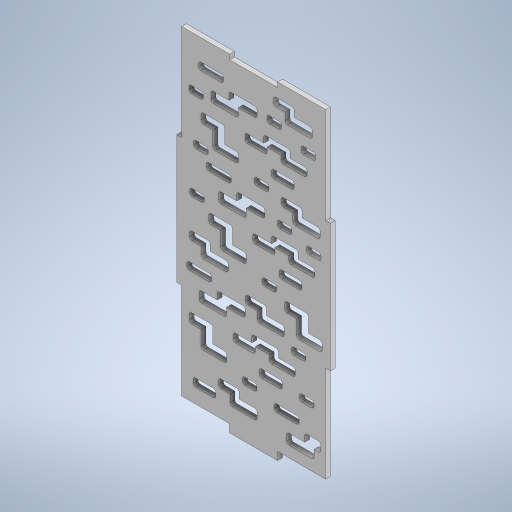
# Autodesk Inventor part: Pièce Ve3
Saved by Autodesk Inventor 2023 (Build 270158000, 158)
## iProperties
Created: 2025-01-14
Part Number: Pièce Ve3
Material: Générique
Document SubType Name: Modeling
Designer: kfadieieva
Density: 1 g/cm^3
Appearance: Par défaut
Author: kfadieieva
Autodesk Inventor part; units mm, degrees
ref_plane "YZ Plane" through (0, 0, 0) normal (1, 0, 0) x (0, 1, 0)
ref_plane "XZ Plane" through (0, 0, 0) normal (0, 1, 0) x (-1, 0, 0)
ref_plane "XY Plane" through (0, 0, 0) normal (0, 0, 1) x (1, 0, 0)
sketch "Esquisse1" plane through (0, 0, 0) normal (0, 0, 1) x (1, 0, 0)
  line L0 (96, 60) -> (96, 139.9775)
  line L1 (0, 140) -> (0, 60)
  line L2 (33, 199.9775) -> (33, 196.9775)
  line L3 (33, 196.9775) -> (63, 196.9775)
  line L4 (63, 196.9775) -> (63, 199.9775)
  line L5 (96, 139.9775) -> (93, 139.9775)
  line L6 (93, 139.9775) -> (93, 199.9775)
  line L7 (96, 60) -> (93, 60)
  line L8 (0, 60) -> (3, 60)
  line L9 (3, 60) -> (3, 0)
  line L10 (0, 140) -> (3, 140)
  line L11 (3, 140) -> (3, 199.9775)
  line L12 (93, 199.9775) -> (63, 199.9775)
  line L13 (33, 199.9775) -> (3, 199.9775)
  line L14 (63, -5) -> (33, -5)
  line L15 (33, -5) -> (33, 0)
  line L16 (3, 0) -> (33, 0)
  line L17 (63, -5) -> (63, 0)
  line L18 (63, 0) -> (93, 0)
  line L19 (93, 0) -> (93, 60)
  point P0 (0, 0)
  point P1 (18, 199.9775)
  dimension "d2" = 33
  dimension "d3" = 33
  dimension "d6" = 3
  dimension "d7" = 3
  dimension "d8" = 3
  dimension "d9" = 3
  dimension "d25" = 33
  dimension "d27" = 60
  dimension "d28" = 90
  dimension "d29" = 90
  dimension "d30" = 90
  dimension "d31" = 90
  dimension "d34" = 90
  dimension "d35" = 90
  dimension "d36" = 90
  dimension "d37" = 90
  dimension "d38" = 90
  dimension "d39" = 5
  dimension "d41" = 90
  dimension "d42" = 90
  dimension "d43" = 90
  dimension "d44" = 96
  dimension "d45" = 199.9775
  constraints: 40 end point, 11 perpendicular, 3 horizontal, 3 parallel, 2 point on line, 2 vertical, 1 midpoint
  measures "d2" distance from line of L0 L4.end
  measures "d3" distance from line of L1 L2.start
  measures "d6" distance of L0.end L5.end
  measures "d7" distance of L1.start L10.end
  measures "d8" distance of L1.end L8.end
  measures "d9" distance of L3.end L4.end
  measures "d25" distance between parallel lines of L15 L1
  measures "d27" distance of L8.end L9.end
  measures "d28" angle of L13 L11
  measures "d29" angle of L2 L13
  measures "d30" angle of L12 L4
  measures "d31" angle of L6 L12
  measures "d34" angle of L16 L9
  measures "d35" angle of L1 L8
  measures "d36" angle of L9 L8
  measures "d37" angle of L10 L1
  measures "d38" angle of L6 L5
  measures "d39" distance of L14.end L15.end
  measures "d41" angle of L14 L15
  measures "d42" angle of L15 L16
  measures "d43" angle of L0 L7
  measures "d44" distance between parallel lines of L0 L1
  measures "d45" distance between parallel lines of L18 L12
extrude "Extrusion1" add sketch "Esquisse1" along normal blind 3
sketch "Esquisse3" plane through (0, 0, 3) normal (0, 0, 1) x (1, 0, 0)
  line L0 (15.2322, 186.7722) -> (27.611, 186.7722)
  line L1 (29.111, 185.2722) -> (29.111, 183.7396)
  line L2 (27.611, 182.2396) -> (15.2322, 182.2396)
  line L3 (13.7322, 183.7396) -> (13.7322, 185.2722)
  line L4 (22.9216, 174.793) -> (32.6723, 174.793)
  line L5 (38.5001, 173.8217) -> (38.5001, 169.8178)
  line L6 (37.0001, 168.3178) -> (22.9216, 168.3178)
  line L7 (21.4216, 169.8178) -> (21.4216, 173.293)
  line L8 (34.1723, 179.8113) -> (48.6555, 179.8113)
  line L9 (50.1555, 178.3113) -> (50.1555, 175.3217)
  line L10 (48.6555, 173.8217) -> (38.5001, 173.8217)
  line L11 (32.6723, 174.793) -> (32.6723, 178.3113)
  line L12 (62.016, 191.143) -> (71.9234, 191.143)
  line L13 (73.4234, 189.643) -> (73.4234, 185.9628)
  line L14 (67.7197, 185.9628) -> (62.016, 185.9628)
  line L15 (60.516, 187.4628) -> (60.516, 189.643)
  line L16 (73.4234, 185.9628) -> (83.1363, 185.9628)
  line L17 (84.6363, 184.4628) -> (84.6363, 181.3113)
  line L18 (83.1363, 179.8113) -> (69.2197, 179.8113)
  line L19 (67.7197, 181.3113) -> (67.7197, 185.9628)
  line L20 (55.8645, 167.1846) -> (69.3764, 167.1846)
  line L21 (70.8764, 165.6846) -> (70.8764, 162.49)
  line L22 (65.2105, 161.5187) -> (56.4689, 161.5187)
  line L23 (54.3645, 162.49) -> (54.3645, 165.6846)
  line L24 (70.8764, 162.49) -> (79.8987, 162.49)
  line L25 (81.3987, 160.99) -> (81.3987, 158.8098)
  line L26 (79.8987, 157.3098) -> (66.7105, 157.3098)
  line L27 (65.2105, 158.8098) -> (65.2105, 161.5187)
  line L28 (44.209, 162.49) -> (54.3645, 162.49)
  line L29 (56.4689, 161.5187) -> (56.4689, 158.8098)
  line L30 (54.9689, 157.3098) -> (44.209, 157.3098)
  line L31 (42.709, 158.8098) -> (42.709, 160.99)
  line L32 (16.6892, 159.8999) -> (28.4608, 159.8999)
  line L33 (29.9608, 158.3999) -> (29.9608, 153.9103)
  line L34 (22.575, 153.9103) -> (16.6892, 153.9103)
  line L35 (15.1892, 155.4103) -> (15.1892, 158.3999)
  line L36 (29.9608, 155.5291) -> (29.9608, 149.5395)
  line L37 (22.575, 147.2732) -> (22.575, 153.9103)
  line L38 (29.9608, 149.5395) -> (37.0001, 149.5395)
  line L39 (38.5001, 148.0395) -> (38.5001, 144.888)
  line L40 (37.0001, 143.388) -> (24.075, 143.388)
  line L41 (22.575, 144.888) -> (22.575, 149.5395)
  line L42 (60.7209, 151.4012) -> (71.8046, 151.4012)
  line L43 (73.3046, 149.9012) -> (73.3046, 147.9638)
  line L44 (71.8046, 146.4638) -> (60.7209, 146.4638)
  line L45 (59.2209, 147.9638) -> (59.2209, 149.9012)
  line L46 (50.0075, 141.672) -> (55.9505, 141.672)
  line L47 (57.4505, 140.172) -> (57.4505, 138.8448)
  line L48 (55.9505, 137.3448) -> (50.0075, 137.3448)
  line L49 (48.5075, 138.8448) -> (48.5075, 140.172)
  arc A0 (15.2322, 186.7722) -> (13.7322, 185.2722) centre (15.2322, 185.2722) ccw
  arc A1 (13.7322, 183.7396) -> (15.2322, 182.2396) centre (15.2322, 183.7396) ccw
  arc A2 (29.111, 185.2722) -> (27.611, 186.7722) centre (27.611, 185.2722) ccw
  arc A3 (27.611, 182.2396) -> (29.111, 183.7396) centre (27.611, 183.7396) ccw
  arc A4 (34.1723, 179.8113) -> (32.6723, 178.3113) centre (34.1723, 178.3113) ccw
  arc A5 (22.9216, 174.793) -> (21.4216, 173.293) centre (22.9216, 173.293) ccw
  arc A6 (21.4216, 169.8178) -> (22.9216, 168.3178) centre (22.9216, 169.8178) ccw
  arc A7 (37.0001, 168.3178) -> (38.5001, 169.8178) centre (37.0001, 169.8178) ccw
  arc A8 (50.1555, 178.3113) -> (48.6555, 179.8113) centre (48.6555, 178.3113) ccw
  arc A9 (48.6555, 173.8217) -> (50.1555, 175.3217) centre (48.6555, 175.3217) ccw
  arc A10 (60.516, 187.4628) -> (62.016, 185.9628) centre (62.016, 187.4628) ccw
  arc A11 (62.016, 191.143) -> (60.516, 189.643) centre (62.016, 189.643) ccw
  arc A12 (73.4234, 189.643) -> (71.9234, 191.143) centre (71.9234, 189.643) ccw
  arc A13 (83.1363, 179.8113) -> (84.6363, 181.3113) centre (83.1363, 181.3113) ccw
  arc A14 (84.6363, 184.4628) -> (83.1363, 185.9628) centre (83.1363, 184.4628) ccw
  arc A15 (67.7197, 181.3113) -> (69.2197, 179.8113) centre (69.2197, 181.3113) ccw
  arc A16 (70.8764, 165.6846) -> (69.3764, 167.1846) centre (69.3764, 165.6846) ccw
  arc A17 (65.2105, 158.8098) -> (66.7105, 157.3098) centre (66.7105, 158.8098) ccw
  arc A18 (81.3987, 160.99) -> (79.8987, 162.49) centre (79.8987, 160.99) ccw
  arc A19 (79.8987, 157.3098) -> (81.3987, 158.8098) centre (79.8987, 158.8098) ccw
  arc A20 (55.8645, 167.1846) -> (54.3645, 165.6846) centre (55.8645, 165.6846) ccw
  arc A21 (44.209, 162.49) -> (42.709, 160.99) centre (44.209, 160.99) ccw
  arc A22 (42.709, 158.8098) -> (44.209, 157.3098) centre (44.209, 158.8098) ccw
  arc A23 (54.9689, 157.3098) -> (56.4689, 158.8098) centre (54.9689, 158.8098) ccw
  arc A24 (60.7209, 151.4012) -> (59.2209, 149.9012) centre (60.7209, 149.9012) ccw
  arc A25 (59.2209, 147.9638) -> (60.7209, 146.4638) centre (60.7209, 147.9638) ccw
  arc A26 (71.8046, 146.4638) -> (73.3046, 147.9638) centre (71.8046, 147.9638) ccw
  arc A27 (73.3046, 149.9012) -> (71.8046, 151.4012) centre (71.8046, 149.9012) ccw
  arc A28 (57.4505, 140.172) -> (55.9505, 141.672) centre (55.9505, 140.172) ccw
  arc A29 (55.9505, 137.3448) -> (57.4505, 138.8448) centre (55.9505, 138.8448) ccw
  arc A30 (48.5075, 138.8448) -> (50.0075, 137.3448) centre (50.0075, 138.8448) ccw
  arc A31 (50.0075, 141.672) -> (48.5075, 140.172) centre (50.0075, 140.172) ccw
  arc A32 (37.0001, 143.388) -> (38.5001, 144.888) centre (37.0001, 144.888) ccw
  arc A33 (38.5001, 148.0395) -> (37.0001, 149.5395) centre (37.0001, 148.0395) ccw
  arc A34 (22.575, 144.888) -> (24.075, 143.388) centre (24.075, 144.888) ccw
  arc A35 (15.1892, 155.4103) -> (16.6892, 153.9103) centre (16.6892, 155.4103) ccw
  arc A36 (16.6892, 159.8999) -> (15.1892, 158.3999) centre (16.6892, 158.3999) ccw
  arc A37 (29.9608, 158.3999) -> (28.4608, 159.8999) centre (28.4608, 158.3999) ccw
  line L50 (20.1228, 134.7776) -> (32.5015, 134.7776)
  line L51 (34.0015, 133.2776) -> (34.0015, 131.7449)
  line L52 (32.5015, 130.2449) -> (20.1228, 130.2449)
  line L53 (18.6228, 131.7449) -> (18.6228, 133.2776)
  line L54 (27.8122, 122.7984) -> (37.5629, 122.7984)
  line L55 (43.3907, 121.8271) -> (43.3907, 117.8231)
  line L56 (41.8907, 116.3231) -> (27.8122, 116.3231)
  line L57 (26.3122, 117.8231) -> (26.3122, 121.2984)
  line L58 (39.0629, 127.8167) -> (53.5461, 127.8167)
  line L59 (55.0461, 126.3167) -> (55.0461, 123.3271)
  line L60 (53.5461, 121.8271) -> (43.3907, 121.8271)
  line L61 (37.5629, 122.7984) -> (37.5629, 126.3167)
  line L62 (66.9065, 139.1484) -> (76.814, 139.1484)
  line L63 (78.314, 137.6484) -> (78.314, 133.9682)
  line L64 (72.6103, 133.9682) -> (66.9065, 133.9682)
  line L65 (65.4065, 135.4682) -> (65.4065, 137.6484)
  line L66 (78.314, 133.9682) -> (88.0269, 133.9682)
  line L67 (89.5269, 132.4682) -> (89.5269, 129.3167)
  line L68 (88.0269, 127.8167) -> (74.1103, 127.8167)
  line L69 (72.6103, 129.3167) -> (72.6103, 133.9682)
  line L70 (60.7551, 115.1899) -> (74.267, 115.1899)
  line L71 (75.767, 113.6899) -> (75.767, 110.4954)
  line L72 (70.1011, 109.5241) -> (61.3595, 109.5241)
  line L73 (59.2551, 110.4954) -> (59.2551, 113.6899)
  line L74 (75.767, 110.4954) -> (84.7893, 110.4954)
  line L75 (86.2893, 108.9954) -> (86.2893, 106.8152)
  line L76 (84.7893, 105.3152) -> (71.6011, 105.3152)
  line L77 (70.1011, 106.8152) -> (70.1011, 109.5241)
  line L78 (49.0996, 110.4954) -> (59.2551, 110.4954)
  line L79 (61.3595, 109.5241) -> (61.3595, 106.8152)
  line L80 (59.8595, 105.3152) -> (49.0996, 105.3152)
  line L81 (47.5996, 106.8152) -> (47.5996, 108.9954)
  line L82 (21.5797, 107.9053) -> (33.3514, 107.9053)
  line L83 (34.8514, 106.4053) -> (34.8514, 101.9156)
  line L84 (27.4656, 101.9156) -> (21.5797, 101.9156)
  line L85 (20.0797, 103.4156) -> (20.0797, 106.4053)
  line L86 (34.8514, 103.5345) -> (34.8514, 97.5448)
  line L87 (27.4656, 95.2785) -> (27.4656, 101.9156)
  line L88 (34.8514, 97.5448) -> (41.8907, 97.5448)
  line L89 (43.3907, 96.0448) -> (43.3907, 92.8933)
  line L90 (41.8907, 91.3933) -> (28.9656, 91.3933)
  line L91 (27.4656, 92.8933) -> (27.4656, 97.5448)
  line L92 (65.6115, 99.4065) -> (76.6952, 99.4065)
  line L93 (78.1952, 97.9065) -> (78.1952, 95.9691)
  line L94 (76.6952, 94.4691) -> (65.6115, 94.4691)
  line L95 (64.1115, 95.9691) -> (64.1115, 97.9065)
  line L96 (54.8981, 89.6774) -> (60.8411, 89.6774)
  line L97 (62.3411, 88.1774) -> (62.3411, 86.8501)
  line L98 (60.8411, 85.3501) -> (54.8981, 85.3501)
  line L99 (53.3981, 86.8501) -> (53.3981, 88.1774)
  arc A38 (20.1228, 134.7776) -> (18.6228, 133.2776) centre (20.1228, 133.2776) ccw
  arc A39 (18.6228, 131.7449) -> (20.1228, 130.2449) centre (20.1228, 131.7449) ccw
  arc A40 (34.0015, 133.2776) -> (32.5015, 134.7776) centre (32.5015, 133.2776) ccw
  arc A41 (32.5015, 130.2449) -> (34.0015, 131.7449) centre (32.5015, 131.7449) ccw
  arc A42 (39.0629, 127.8167) -> (37.5629, 126.3167) centre (39.0629, 126.3167) ccw
  arc A43 (27.8122, 122.7984) -> (26.3122, 121.2984) centre (27.8122, 121.2984) ccw
  arc A44 (26.3122, 117.8231) -> (27.8122, 116.3231) centre (27.8122, 117.8231) ccw
  arc A45 (41.8907, 116.3231) -> (43.3907, 117.8231) centre (41.8907, 117.8231) ccw
  arc A46 (55.0461, 126.3167) -> (53.5461, 127.8167) centre (53.5461, 126.3167) ccw
  arc A47 (53.5461, 121.8271) -> (55.0461, 123.3271) centre (53.5461, 123.3271) ccw
  arc A48 (65.4065, 135.4682) -> (66.9065, 133.9682) centre (66.9065, 135.4682) ccw
  arc A49 (66.9065, 139.1484) -> (65.4065, 137.6484) centre (66.9065, 137.6484) ccw
  arc A50 (78.314, 137.6484) -> (76.814, 139.1484) centre (76.814, 137.6484) ccw
  arc A51 (88.0269, 127.8167) -> (89.5269, 129.3167) centre (88.0269, 129.3167) ccw
  arc A52 (89.5269, 132.4682) -> (88.0269, 133.9682) centre (88.0269, 132.4682) ccw
  arc A53 (72.6103, 129.3167) -> (74.1103, 127.8167) centre (74.1103, 129.3167) ccw
  arc A54 (75.767, 113.6899) -> (74.267, 115.1899) centre (74.267, 113.6899) ccw
  arc A55 (70.1011, 106.8152) -> (71.6011, 105.3152) centre (71.6011, 106.8152) ccw
  arc A56 (86.2893, 108.9954) -> (84.7893, 110.4954) centre (84.7893, 108.9954) ccw
  arc A57 (84.7893, 105.3152) -> (86.2893, 106.8152) centre (84.7893, 106.8152) ccw
  arc A58 (60.7551, 115.1899) -> (59.2551, 113.6899) centre (60.7551, 113.6899) ccw
  arc A59 (49.0996, 110.4954) -> (47.5996, 108.9954) centre (49.0996, 108.9954) ccw
  arc A60 (47.5996, 106.8152) -> (49.0996, 105.3152) centre (49.0996, 106.8152) ccw
  arc A61 (59.8595, 105.3152) -> (61.3595, 106.8152) centre (59.8595, 106.8152) ccw
  arc A62 (65.6115, 99.4065) -> (64.1115, 97.9065) centre (65.6115, 97.9065) ccw
  arc A63 (64.1115, 95.9691) -> (65.6115, 94.4691) centre (65.6115, 95.9691) ccw
  arc A64 (76.6952, 94.4691) -> (78.1952, 95.9691) centre (76.6952, 95.9691) ccw
  arc A65 (78.1952, 97.9065) -> (76.6952, 99.4065) centre (76.6952, 97.9065) ccw
  arc A66 (62.3411, 88.1774) -> (60.8411, 89.6774) centre (60.8411, 88.1774) ccw
  arc A67 (60.8411, 85.3501) -> (62.3411, 86.8501) centre (60.8411, 86.8501) ccw
  arc A68 (53.3981, 86.8501) -> (54.8981, 85.3501) centre (54.8981, 86.8501) ccw
  arc A69 (54.8981, 89.6774) -> (53.3981, 88.1774) centre (54.8981, 88.1774) ccw
  arc A70 (41.8907, 91.3933) -> (43.3907, 92.8933) centre (41.8907, 92.8933) ccw
  arc A71 (43.3907, 96.0448) -> (41.8907, 97.5448) centre (41.8907, 96.0448) ccw
  arc A72 (27.4656, 92.8933) -> (28.9656, 91.3933) centre (28.9656, 92.8933) ccw
  arc A73 (20.0797, 103.4156) -> (21.5797, 101.9156) centre (21.5797, 103.4156) ccw
  arc A74 (21.5797, 107.9053) -> (20.0797, 106.4053) centre (21.5797, 106.4053) ccw
  arc A75 (34.8514, 106.4053) -> (33.3514, 107.9053) centre (33.3514, 106.4053) ccw
  line L100 (7.859, 75.0609) -> (20.2378, 75.0609)
  line L101 (21.7378, 73.5609) -> (21.7378, 72.0282)
  line L102 (20.2378, 70.5282) -> (7.859, 70.5282)
  line L103 (6.359, 72.0282) -> (6.359, 73.5609)
  line L104 (15.5484, 63.0817) -> (25.2992, 63.0817)
  line L105 (31.1269, 62.1104) -> (31.1269, 58.1064)
  line L106 (29.6269, 56.6064) -> (15.5484, 56.6064)
  line L107 (14.0484, 58.1064) -> (14.0484, 61.5817)
  line L108 (26.7992, 68.1) -> (41.2824, 68.1)
  line L109 (42.7824, 66.6) -> (42.7824, 63.6104)
  line L110 (41.2824, 62.1104) -> (31.1269, 62.1104)
  line L111 (25.2992, 63.0817) -> (25.2992, 66.6)
  line L112 (44.5787, 75.1578) -> (54.4861, 75.1578)
  line L113 (55.9861, 73.6578) -> (55.9861, 69.9776)
  line L114 (50.2824, 69.9776) -> (44.5787, 69.9776)
  line L115 (43.0787, 71.4776) -> (43.0787, 73.6578)
  line L116 (55.9861, 69.9776) -> (65.699, 69.9776)
  line L117 (67.199, 68.4776) -> (67.199, 65.3261)
  line L118 (65.699, 63.8261) -> (51.7824, 63.8261)
  line L119 (50.2824, 65.3261) -> (50.2824, 69.9776)
  line L120 (48.4913, 55.4733) -> (62.0032, 55.4733)
  line L121 (63.5032, 53.9733) -> (63.5032, 50.7787)
  line L122 (57.8373, 49.8074) -> (49.0957, 49.8074)
  line L123 (46.9913, 50.7787) -> (46.9913, 53.9733)
  line L124 (63.5032, 50.7787) -> (72.5255, 50.7787)
  line L125 (74.0255, 49.2787) -> (74.0255, 47.0985)
  line L126 (72.5255, 45.5985) -> (59.3373, 45.5985)
  line L127 (57.8373, 47.0985) -> (57.8373, 49.8074)
  line L128 (36.8358, 50.7787) -> (46.9913, 50.7787)
  line L129 (49.0957, 49.8074) -> (49.0957, 47.0985)
  line L130 (47.5957, 45.5985) -> (36.8358, 45.5985)
  line L131 (35.3358, 47.0985) -> (35.3358, 49.2787)
  line L132 (9.316, 48.1886) -> (21.0877, 48.1886)
  line L133 (22.5877, 46.6886) -> (22.5877, 42.199)
  line L134 (15.2018, 42.199) -> (9.316, 42.199)
  line L135 (7.816, 43.699) -> (7.816, 46.6886)
  line L136 (22.5877, 43.8178) -> (22.5877, 37.8282)
  line L137 (15.2018, 35.5619) -> (15.2018, 42.199)
  line L138 (22.5877, 37.8282) -> (29.6269, 37.8282)
  line L139 (31.1269, 36.3282) -> (31.1269, 33.1767)
  line L140 (29.6269, 31.6767) -> (16.7018, 31.6767)
  line L141 (15.2018, 33.1767) -> (15.2018, 37.8282)
  line L142 (53.3477, 39.6898) -> (64.4314, 39.6898)
  line L143 (65.9314, 38.1898) -> (65.9314, 36.2524)
  line L144 (64.4314, 34.7524) -> (53.3477, 34.7524)
  line L145 (51.8477, 36.2524) -> (51.8477, 38.1898)
  line L146 (42.6343, 29.9607) -> (48.5773, 29.9607)
  line L147 (50.0773, 28.4607) -> (50.0773, 27.1335)
  line L148 (48.5773, 25.6335) -> (42.6343, 25.6335)
  line L149 (41.1343, 27.1335) -> (41.1343, 28.4607)
  arc A76 (7.859, 75.0609) -> (6.359, 73.5609) centre (7.859, 73.5609) ccw
  arc A77 (6.359, 72.0282) -> (7.859, 70.5282) centre (7.859, 72.0282) ccw
  arc A78 (21.7378, 73.5609) -> (20.2378, 75.0609) centre (20.2378, 73.5609) ccw
  arc A79 (20.2378, 70.5282) -> (21.7378, 72.0282) centre (20.2378, 72.0282) ccw
  arc A80 (26.7992, 68.1) -> (25.2992, 66.6) centre (26.7992, 66.6) ccw
  arc A81 (15.5484, 63.0817) -> (14.0484, 61.5817) centre (15.5484, 61.5817) ccw
  arc A82 (14.0484, 58.1064) -> (15.5484, 56.6064) centre (15.5484, 58.1064) ccw
  arc A83 (29.6269, 56.6064) -> (31.1269, 58.1064) centre (29.6269, 58.1064) ccw
  arc A84 (42.7824, 66.6) -> (41.2824, 68.1) centre (41.2824, 66.6) ccw
  arc A85 (41.2824, 62.1104) -> (42.7824, 63.6104) centre (41.2824, 63.6104) ccw
  arc A86 (43.0787, 71.4776) -> (44.5787, 69.9776) centre (44.5787, 71.4776) ccw
  arc A87 (44.5787, 75.1578) -> (43.0787, 73.6578) centre (44.5787, 73.6578) ccw
  arc A88 (55.9861, 73.6578) -> (54.4861, 75.1578) centre (54.4861, 73.6578) ccw
  arc A89 (65.699, 63.8261) -> (67.199, 65.3261) centre (65.699, 65.3261) ccw
  arc A90 (67.199, 68.4776) -> (65.699, 69.9776) centre (65.699, 68.4776) ccw
  arc A91 (50.2824, 65.3261) -> (51.7824, 63.8261) centre (51.7824, 65.3261) ccw
  arc A92 (63.5032, 53.9733) -> (62.0032, 55.4733) centre (62.0032, 53.9733) ccw
  arc A93 (57.8373, 47.0985) -> (59.3373, 45.5985) centre (59.3373, 47.0985) ccw
  arc A94 (74.0255, 49.2787) -> (72.5255, 50.7787) centre (72.5255, 49.2787) ccw
  arc A95 (72.5255, 45.5985) -> (74.0255, 47.0985) centre (72.5255, 47.0985) ccw
  arc A96 (48.4913, 55.4733) -> (46.9913, 53.9733) centre (48.4913, 53.9733) ccw
  arc A97 (36.8358, 50.7787) -> (35.3358, 49.2787) centre (36.8358, 49.2787) ccw
  arc A98 (35.3358, 47.0985) -> (36.8358, 45.5985) centre (36.8358, 47.0985) ccw
  arc A99 (47.5957, 45.5985) -> (49.0957, 47.0985) centre (47.5957, 47.0985) ccw
  arc A100 (53.3477, 39.6898) -> (51.8477, 38.1898) centre (53.3477, 38.1898) ccw
  arc A101 (51.8477, 36.2524) -> (53.3477, 34.7524) centre (53.3477, 36.2524) ccw
  arc A102 (64.4314, 34.7524) -> (65.9314, 36.2524) centre (64.4314, 36.2524) ccw
  arc A103 (65.9314, 38.1898) -> (64.4314, 39.6898) centre (64.4314, 38.1898) ccw
  arc A104 (50.0773, 28.4607) -> (48.5773, 29.9607) centre (48.5773, 28.4607) ccw
  arc A105 (48.5773, 25.6335) -> (50.0773, 27.1335) centre (48.5773, 27.1335) ccw
  arc A106 (41.1343, 27.1335) -> (42.6343, 25.6335) centre (42.6343, 27.1335) ccw
  arc A107 (42.6343, 29.9607) -> (41.1343, 28.4607) centre (42.6343, 28.4607) ccw
  arc A108 (29.6269, 31.6767) -> (31.1269, 33.1767) centre (29.6269, 33.1767) ccw
  arc A109 (31.1269, 36.3282) -> (29.6269, 37.8282) centre (29.6269, 36.3282) ccw
  arc A110 (15.2018, 33.1767) -> (16.7018, 31.6767) centre (16.7018, 33.1767) ccw
  arc A111 (7.816, 43.699) -> (9.316, 42.199) centre (9.316, 43.699) ccw
  arc A112 (9.316, 48.1886) -> (7.816, 46.6886) centre (9.316, 46.6886) ccw
  arc A113 (22.5877, 46.6886) -> (21.0877, 48.1886) centre (21.0877, 46.6886) ccw
  line L150 (62.5345, 25.4266) -> (74.9132, 25.4266)
  line L151 (76.4132, 23.9266) -> (76.4132, 22.3939)
  line L152 (74.9132, 20.8939) -> (62.5345, 20.8939)
  line L153 (61.0345, 22.3939) -> (61.0345, 23.9266)
  line L154 (70.2239, 13.4474) -> (79.9746, 13.4474)
  line L155 (85.8024, 12.4761) -> (85.8024, 8.4721)
  line L156 (84.3024, 6.9721) -> (70.2239, 6.9721)
  line L157 (68.7239, 8.4721) -> (68.7239, 11.9474)
  line L158 (79.9746, 13.4474) -> (79.9746, 16.9657)
  line L159 (9.5387, 92.4703) -> (19.4461, 92.4703)
  line L160 (20.9461, 90.9703) -> (20.9461, 87.2901)
  line L161 (15.2424, 87.2901) -> (9.5387, 87.2901)
  line L162 (8.0387, 88.7901) -> (8.0387, 90.9703)
  line L163 (20.9461, 87.2901) -> (30.659, 87.2901)
  line L164 (32.159, 85.7901) -> (32.159, 82.6386)
  line L165 (30.659, 81.1386) -> (16.7424, 81.1386)
  line L166 (15.2424, 82.6386) -> (15.2424, 87.2901)
  line L167 (69.0763, 83.9073) -> (80.848, 83.9073)
  line L168 (82.348, 82.4073) -> (82.348, 77.9177)
  line L169 (74.9621, 77.9177) -> (69.0763, 77.9177)
  line L170 (67.5763, 79.4177) -> (67.5763, 82.4073)
  line L171 (82.348, 79.5365) -> (82.348, 73.5469)
  line L172 (74.9621, 71.2806) -> (74.9621, 77.9177)
  line L173 (82.348, 73.5469) -> (89.3872, 73.5469)
  line L174 (90.8872, 72.0469) -> (90.8872, 68.8954)
  line L175 (89.3872, 67.3954) -> (76.4621, 67.3954)
  line L176 (74.9621, 68.8954) -> (74.9621, 73.5469)
  line L177 (11.7943, 14.1137) -> (22.878, 14.1137)
  line L178 (24.378, 12.6137) -> (24.378, 10.6763)
  line L179 (22.878, 9.1763) -> (11.7943, 9.1763)
  line L180 (10.2943, 10.6763) -> (10.2943, 12.6137)
  line L181 (78.3166, 38.6119) -> (84.2595, 38.6119)
  line L182 (85.7595, 37.1119) -> (85.7595, 35.7846)
  line L183 (84.2595, 34.2846) -> (78.3166, 34.2846)
  line L184 (76.8166, 35.7846) -> (76.8166, 37.1119)
  arc A114 (62.5345, 25.4266) -> (61.0345, 23.9266) centre (62.5345, 23.9266) ccw
  arc A115 (61.0345, 22.3939) -> (62.5345, 20.8939) centre (62.5345, 22.3939) ccw
  arc A116 (76.4132, 23.9266) -> (74.9132, 25.4266) centre (74.9132, 23.9266) ccw
  arc A117 (74.9132, 20.8939) -> (76.4132, 22.3939) centre (74.9132, 22.3939) ccw
  arc A118 (81.4746, 18.4657) -> (79.9746, 16.9657) centre (81.4746, 16.9657) ccw
  arc A119 (70.2239, 13.4474) -> (68.7239, 11.9474) centre (70.2239, 11.9474) ccw
  arc A120 (68.7239, 8.4721) -> (70.2239, 6.9721) centre (70.2239, 8.4721) ccw
  arc A121 (84.3024, 6.9721) -> (85.8024, 8.4721) centre (84.3024, 8.4721) ccw
  arc A122 (8.0387, 88.7901) -> (9.5387, 87.2901) centre (9.5387, 88.7901) ccw
  arc A123 (9.5387, 92.4703) -> (8.0387, 90.9703) centre (9.5387, 90.9703) ccw
  arc A124 (20.9461, 90.9703) -> (19.4461, 92.4703) centre (19.4461, 90.9703) ccw
  arc A125 (30.659, 81.1386) -> (32.159, 82.6386) centre (30.659, 82.6386) ccw
  arc A126 (32.159, 85.7901) -> (30.659, 87.2901) centre (30.659, 85.7901) ccw
  arc A127 (15.2424, 82.6386) -> (16.7424, 81.1386) centre (16.7424, 82.6386) ccw
  arc A128 (11.7943, 14.1137) -> (10.2943, 12.6137) centre (11.7943, 12.6137) ccw
  arc A129 (10.2943, 10.6763) -> (11.7943, 9.1763) centre (11.7943, 10.6763) ccw
  arc A130 (22.878, 9.1763) -> (24.378, 10.6763) centre (22.878, 10.6763) ccw
  arc A131 (24.378, 12.6137) -> (22.878, 14.1137) centre (22.878, 12.6137) ccw
  arc A132 (85.7595, 37.1119) -> (84.2595, 38.6119) centre (84.2595, 37.1119) ccw
  arc A133 (84.2595, 34.2846) -> (85.7595, 35.7846) centre (84.2595, 35.7846) ccw
  arc A134 (76.8166, 35.7846) -> (78.3166, 34.2846) centre (78.3166, 35.7846) ccw
  arc A135 (78.3166, 38.6119) -> (76.8166, 37.1119) centre (78.3166, 37.1119) ccw
  arc A136 (89.3872, 67.3954) -> (90.8872, 68.8954) centre (89.3872, 68.8954) ccw
  arc A137 (90.8872, 72.0469) -> (89.3872, 73.5469) centre (89.3872, 72.0469) ccw
  arc A138 (74.9621, 68.8954) -> (76.4621, 67.3954) centre (76.4621, 68.8954) ccw
  arc A139 (67.5763, 79.4177) -> (69.0763, 77.9177) centre (69.0763, 79.4177) ccw
  arc A140 (69.0763, 83.9073) -> (67.5763, 82.4073) centre (69.0763, 82.4073) ccw
  arc A141 (82.348, 82.4073) -> (80.848, 83.9073) centre (80.848, 82.4073) ccw
  line L185 (27.6073, 21.4563) -> (37.5148, 21.4563)
  line L186 (39.0148, 19.9563) -> (39.0148, 16.2761)
  line L187 (33.3111, 16.2761) -> (27.6073, 16.2761)
  line L188 (26.1073, 17.7761) -> (26.1073, 19.9563)
  line L189 (39.0148, 16.2761) -> (48.7277, 16.2761)
  line L190 (50.2277, 14.7761) -> (50.2277, 11.6246)
  line L191 (48.7277, 10.1246) -> (34.8111, 10.1246)
  line L192 (33.3111, 11.6246) -> (33.3111, 16.2761)
  line L193 (9.6709, 115.6112) -> (15.6139, 115.6112)
  line L194 (17.1139, 114.1112) -> (17.1139, 112.784)
  line L195 (15.6139, 111.284) -> (9.6709, 111.284)
  line L196 (8.1709, 112.784) -> (8.1709, 114.1112)
  arc A142 (-19.1764, 17.0855) -> (-19.2195, 17.0849) centre (-19.1764, 15.5855) ccw
  arc A143 (26.1073, 17.7761) -> (27.6073, 16.2761) centre (27.6073, 17.7761) ccw
  arc A144 (27.6073, 21.4563) -> (26.1073, 19.9563) centre (27.6073, 19.9563) ccw
  arc A145 (39.0148, 19.9563) -> (37.5148, 21.4563) centre (37.5148, 19.9563) ccw
  arc A146 (48.7277, 10.1246) -> (50.2277, 11.6246) centre (48.7277, 11.6246) ccw
  arc A147 (50.2277, 14.7761) -> (48.7277, 16.2761) centre (48.7277, 14.7761) ccw
  arc A148 (33.3111, 11.6246) -> (34.8111, 10.1246) centre (34.8111, 11.6246) ccw
  arc A149 (17.1139, 114.1112) -> (15.6139, 115.6112) centre (15.6139, 114.1112) ccw
  arc A150 (15.6139, 111.284) -> (17.1139, 112.784) centre (15.6139, 112.784) ccw
  arc A151 (8.1709, 112.784) -> (9.6709, 111.284) centre (9.6709, 112.784) ccw
  arc A152 (9.6709, 115.6112) -> (8.1709, 114.1112) centre (9.6709, 114.1112) ccw
  line L197 (88.5113, 12.4761) -> (85.8024, 12.4761)
  line L198 (81.4746, 18.4657) -> (88.5113, 18.4657)
  line L199 (90.0113, 16.9657) -> (90.0113, 13.9761)
  arc A153 (88.5113, 12.4761) -> (90.0113, 13.9761) centre (88.5113, 13.9761) ccw
  arc A154 (90.0113, 16.9657) -> (88.5113, 18.4657) centre (88.5113, 16.9657) ccw
  line L200 (64.4612, 125.6561) -> (70.4042, 125.6561)
  arc A155 (71.9042, 124.1561) -> (70.4042, 125.6561) centre (70.4042, 124.1561) ccw
  arc A156 (64.4612, 125.6561) -> (62.9612, 124.1561) centre (64.4612, 124.1561) ccw
  line L201 (71.9042, 124.1561) -> (71.9042, 122.8289)
  arc A157 (62.9612, 122.8289) -> (64.4612, 121.3289) centre (64.4612, 122.8289) ccw
  line L202 (70.4042, 121.3289) -> (64.4612, 121.3289)
  arc A158 (70.4042, 121.3289) -> (71.9042, 122.8289) centre (70.4042, 122.8289) ccw
  line L203 (62.9612, 122.8289) -> (62.9612, 124.1561)
  line L204 (82.6873, 120.6683) -> (88.6303, 120.6683)
  arc A159 (90.1303, 119.1683) -> (88.6303, 120.6683) centre (88.6303, 119.1683) ccw
  arc A160 (82.6873, 120.6683) -> (81.1873, 119.1683) centre (82.6873, 119.1683) ccw
  line L205 (90.1303, 119.1683) -> (90.1303, 117.8411)
  arc A161 (81.1873, 117.8411) -> (82.6873, 116.3411) centre (82.6873, 117.8411) ccw
  line L206 (88.6303, 116.3411) -> (82.6873, 116.3411)
  arc A162 (88.6303, 116.3411) -> (90.1303, 117.8411) centre (88.6303, 117.8411) ccw
  line L207 (81.1873, 117.8411) -> (81.1873, 119.1683)
  line L208 (79.2329, 173.1612) -> (85.1759, 173.1612)
  arc A163 (86.6759, 171.6612) -> (85.1759, 173.1612) centre (85.1759, 171.6612) ccw
  arc A164 (79.2329, 173.1612) -> (77.7329, 171.6612) centre (79.2329, 171.6612) ccw
  line L209 (86.6759, 171.6612) -> (86.6759, 170.3339)
  arc A165 (77.7329, 170.3339) -> (79.2329, 168.8339) centre (79.2329, 170.3339) ccw
  line L210 (85.1759, 168.8339) -> (79.2329, 168.8339)
  arc A166 (85.1759, 168.8339) -> (86.6759, 170.3339) centre (85.1759, 170.3339) ccw
  line L211 (77.7329, 170.3339) -> (77.7329, 171.6612)
  line L212 (57.9194, 179.1508) -> (63.8624, 179.1508)
  arc A167 (65.3624, 177.6508) -> (63.8624, 179.1508) centre (63.8624, 177.6508) ccw
  arc A168 (57.9194, 179.1508) -> (56.4194, 177.6508) centre (57.9194, 177.6508) ccw
  line L213 (65.3624, 177.6508) -> (65.3624, 176.3235)
  arc A169 (56.4194, 176.3235) -> (57.9194, 174.8235) centre (57.9194, 176.3235) ccw
  line L214 (63.8624, 174.8235) -> (57.9194, 174.8235)
  arc A170 (63.8624, 174.8235) -> (65.3624, 176.3235) centre (63.8624, 176.3235) ccw
  line L215 (56.4194, 176.3235) -> (56.4194, 177.6508)
  line L216 (12.1274, 142.7275) -> (18.0703, 142.7275)
  arc A171 (19.5703, 141.2275) -> (18.0703, 142.7275) centre (18.0703, 141.2275) ccw
  arc A172 (12.1274, 142.7275) -> (10.6274, 141.2275) centre (12.1274, 141.2275) ccw
  line L217 (19.5703, 141.2275) -> (19.5703, 139.9002)
  arc A173 (10.6274, 139.9002) -> (12.1274, 138.4002) centre (12.1274, 139.9002) ccw
  line L218 (18.0703, 138.4002) -> (12.1274, 138.4002)
  arc A174 (18.0703, 138.4002) -> (19.5703, 139.9002) centre (18.0703, 139.9002) ccw
  line L219 (10.6274, 139.9002) -> (10.6274, 141.2275)
  line L220 (9.1438, 171.1592) -> (15.0868, 171.1592)
  arc A175 (16.5868, 169.6592) -> (15.0868, 171.1592) centre (15.0868, 169.6592) ccw
  arc A176 (9.1438, 171.1592) -> (7.6438, 169.6592) centre (9.1438, 169.6592) ccw
  line L221 (16.5868, 169.6592) -> (16.5868, 168.3319)
  arc A177 (7.6438, 168.3319) -> (9.1438, 166.8319) centre (9.1438, 168.3319) ccw
  line L222 (15.0868, 166.8319) -> (9.1438, 166.8319)
  arc A178 (15.0868, 166.8319) -> (16.5868, 168.3319) centre (15.0868, 168.3319) ccw
  line L223 (7.6438, 168.3319) -> (7.6438, 169.6592)
  line L224 (73.2982, 61.4499) -> (79.2412, 61.4499)
  arc A179 (80.7412, 59.9499) -> (79.2412, 61.4499) centre (79.2412, 59.9499) ccw
  arc A180 (73.2982, 61.4499) -> (71.7982, 59.9499) centre (73.2982, 59.9499) ccw
  line L225 (80.7412, 59.9499) -> (80.7412, 58.6226)
  arc A181 (71.7982, 58.6226) -> (73.2982, 57.1226) centre (73.2982, 58.6226) ccw
  line L226 (79.2412, 57.1226) -> (73.2982, 57.1226)
  arc A182 (79.2412, 57.1226) -> (80.7412, 58.6226) centre (79.2412, 58.6226) ccw
  line L227 (71.7982, 58.6226) -> (71.7982, 59.9499)
  point P0 (0, 0)
  point P1 (84.6363, 179.8113)
  point P2 (42.709, 162.49)
  point P3 (56.4689, 157.3098)
  point P4 (38.5001, 143.388)
  point P5 (89.5269, 127.8167)
  point P6 (47.5996, 110.4954)
  point P7 (61.3595, 105.3152)
  point P8 (43.3907, 91.3933)
  point P9 (67.199, 63.8261)
  point P10 (35.3358, 50.7787)
  point P11 (49.0957, 45.5985)
  point P12 (31.1269, 31.6767)
  point P13 (32.159, 81.1386)
  point P14 (90.8872, 67.3954)
  point P15 (50.2277, 10.1246)
  point P16 (90.0113, 12.4761)
  point P17 (90.0113, 18.4657)
  dimension "d12" = 1.5
  dimension "d13" = 1.5
  dimension "d14" = 1.5
  dimension "d15" = 1.5
  dimension "d16" = 1.5
  dimension "d17" = 1.5
  constraints: 456 end point, 366 point on circle, 364 tangent, 183 centre point, 149 equal radius, 113 parallel, 55 horizontal, 54 perpendicular, 49 point on line, 1 vertical
  measures "d12" radius of A0
  measures "d13" radius of A38
  measures "d14" radius of A76
  measures "d15" radius of A114
  measures "d16" radius of A142
  measures "d17" radius of A153
extrude "Extrusion2" cut sketch "Esquisse3" against normal blind 10
